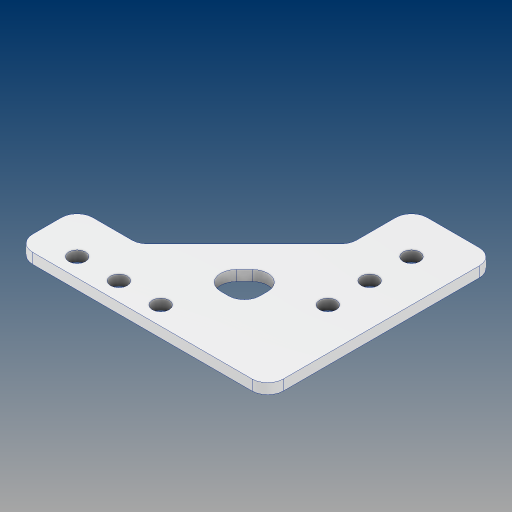
# Autodesk Inventor part: ELEV_005_SUPBRK1
Saved by Autodesk Inventor 2024.3 (Build 283343000, 343)
## iProperties
Created: 2024-11-25
Part Number: ELEV_005_SUPBRK1
Material: Aluminum 6061
Document SubType Name: Modeling
Designer: Kenji
Density: 2.7 g/cm^3
Appearance: Aluminum - Flat
Author: Kenji
Autodesk Inventor part; units mm, degrees
ref_plane "YZ Plane" through (0, 0, 0) normal (1, 0, 0) x (0, 1, 0)
ref_plane "XZ Plane" through (0, 0, 0) normal (0, 1, 0) x (-1, 0, 0)
ref_plane "XY Plane" through (0, 0, 0) normal (0, 0, 1) x (1, 0, 0)
sketch "Sketch1" plane through (0, 0, 0) normal (0, 1, 0) x (-1, 0, 0)
  line L0 (0, 0) -> (15.875, 0) construction
  line L1 (20.6375, -76.2) -> (4.7625, -76.2)
  line L2 (0, -71.4375) -> (0, -11.8745)
  line L3 (30.1625, -25.4) -> (76.2, -25.4) construction
  line L4 (76.2, -20.6375) -> (76.2, -11.8745)
  line L5 (71.4375, -7.112) -> (4.7625, -7.112)
  line L6 (25.4, -76.2) -> (25.4, -30.1625) construction
  arc A0 (30.1625, -25.4) -> (25.4, -30.1625) centre (30.1625, -30.1625) ccw construction
  arc A1 (0, -71.4375) -> (4.7625, -76.2) centre (4.7625, -71.4375) ccw
  arc A2 (76.2, -11.8745) -> (71.4375, -7.112) centre (71.4375, -11.8745) ccw
  arc A3 (4.7625, -7.112) -> (0, -11.8745) centre (4.7625, -11.8745) ccw
  circle A4 centre (12.7, -38.1) radius 2.54
  circle A5 centre (12.7, -50.8) radius 2.54
  circle A6 centre (12.7, -63.5) radius 2.54
  circle A7 centre (63.5, -12.7) radius 2.54
  circle A8 centre (50.8, -12.7) radius 2.54
  circle A9 centre (38.1, -12.7) radius 2.54
  line L7 (76.2, -12.7) -> (0, -12.7) construction
  line L8 (12.7, -7.112) -> (12.7, -76.2) construction
  line L9 (61.7039, -14.4961) -> (14.4961, -61.7039) construction
  line L10 (56.1403, -26.7949) -> (26.7949, -56.1403)
  line L11 (71.4375, -25.4) -> (59.5079, -25.4)
  line L12 (25.4, -59.5079) -> (25.4, -71.4375)
  arc A10 (71.4375, -25.4) -> (76.2, -20.6375) centre (71.4375, -20.6375) ccw
  arc A11 (20.6375, -76.2) -> (25.4, -71.4375) centre (20.6375, -71.4375) ccw
  arc A12 (59.5079, -25.4) -> (56.1403, -26.7949) centre (59.5079, -30.1625) ccw
  arc A13 (26.7949, -56.1403) -> (25.4, -59.5079) centre (30.1625, -59.5079) ccw
  line L13 (35.9347, -33.5301) -> (33.5301, -35.9347)
  line L14 (25.4, -32.5671) -> (25.4, -30.1625)
  line L15 (32.5671, -25.4) -> (30.1625, -25.4)
  arc A14 (30.1625, -25.4) -> (25.4, -30.1625) centre (30.1625, -30.1625) ccw
  arc A15 (35.9347, -33.5301) -> (32.5671, -25.4) centre (32.5671, -30.1625) ccw
  arc A16 (25.4, -32.5671) -> (33.5301, -35.9347) centre (30.1625, -32.5671) ccw
  point P0 (25.4, -76.2)
  point P1 (0, -76.2)
  point P2 (38.1, -12.7)
  point P3 (57.5352, -25.4)
  point P4 (25.4, -57.5352)
  point P5 (44.0648, -25.4)
  point P6 (25.4, -44.0648)
  dimension "d1" = 76.2
  dimension "d2" = 25.4
  dimension "d5" = 4.7625
  dimension "d8" = 5.08
  dimension "d10" = 12.7
  dimension "d11" = 12.7
  dimension "d14" = 12.7
  dimension "d15" = 12.7
  dimension "d18" = 66.675
  dimension "d20" = 25.4
  dimension "d21" = 38.1
  dimension "d22" = 18.288
  dimension "d23" = 38.1
  dimension "d24" = 12.7
  dimension "d25" = 12.7
  dimension "d27" = 4.7625
  dimension "d28" = 4.7625
  dimension "d29" = 4.7625
  dimension "d30" = 4.7625
  constraints: 32 end point, 31 point on line, 22 point on circle, 22 tangent, 15 centre point, 10 equal radius, 5 parallel, 4 perpendicular, 3 horizontal, 3 midpoint, 2 collinear, 2 vertical, 1 coincident, 1 concentric, 8 other
  measures "d1" distance between parallel lines of L1 L0
  measures "d2" distance of point (25.4, -76.2) point (0, -76.2)
  measures "d5" radius of A0
  measures "d8" diameter of A4
  measures "d10" distance of point (12.7, -38.1) A5.centre
  measures "d11" distance of point (12.7, -63.5) A5.centre
  measures "d14" distance of A8.centre point (63.5, -12.7)
  measures "d15" distance of A9.centre A8.centre
  measures "d18" distance of L5.start L5.end
  measures "d20" distance from line of L0.start L3
  measures "d21" vertical distance of L0.start point (12.7, -38.1)
  measures "d22" distance between parallel lines of L3 L5
  measures "d23" distance from line of L2 A9.centre
  measures "d24" distance from line of L0.start L7
  measures "d25" distance between parallel lines of L2 L8
  measures "d27" distance between parallel lines of L9 L10
  measures "d28" radius of A10
  measures "d29" distance between parallel lines of L9 L13
  measures "d30" radius of A15
extrude "Extrusion2" add sketch "Sketch1" along normal blind 3.175 contours L1 A1 L2 A3 L5 A2 L4 A10 L11 A12 L10 A13 L12 A11 | L13 A16 L14 A14 L15 A15
extrude "Extrusion3" cut sketch "Sketch1" along normal through all contours L13 A16 L14 A14 L15 A15
body "Solid2"
